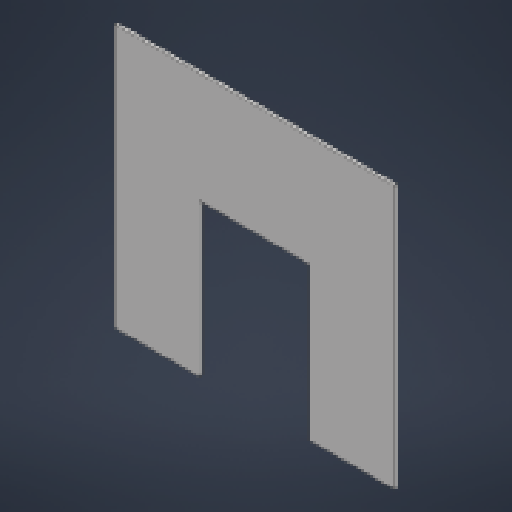
# Autodesk Inventor part: второй верх
Saved by Autodesk Inventor 2026.2 (Build 302298000, 298)
## iProperties
Created: 2025-11-21
Part Number: второй верх
Material: Типовые
Document SubType Name: Modeling
Designer: Phantom
Density: 1 g/cm^3
Appearance: По умолчанию
Author: Phantom
Autodesk Inventor part; units mm, degrees
ref_plane "YZ Plane" through (0, 0, 0) normal (1, 0, 0) x (0, 1, 0)
ref_plane "XZ Plane" through (0, 0, 0) normal (0, 1, 0) x (-1, 0, 0)
ref_plane "XY Plane" through (0, 0, 0) normal (0, 0, 1) x (1, 0, 0)
sketch "Эскиз1" plane through (0, 0, 0) normal (0, 0, 1) x (1, 0, 0)
  line L0 (-202.5, -190) -> (202.5, -190)
  line L1 (202.5, -190) -> (202.5, 190)
  line L2 (202.5, 190) -> (-202.5, 190)
  line L3 (-202.5, 190) -> (-202.5, -190)
  line L4 (-202.5, -190) -> (202.5, 190) construction
  line L5 (202.5, -190) -> (-202.5, 190) construction
  point P0 (0, 0)
  dimension "d0" = 405
  dimension "d1" = 380
  constraints: 12 end point, 2 midpoint, 2 parallel, 1 horizontal, 1 perpendicular
  measures "d0" distance of L2.end L1.end
  measures "d1" distance of L1.end L0.end
extrude "Выдавливание1" add sketch "Эскиз1" along normal blind 4
sketch "Эскиз2" plane through (0, 0, 4) normal (0, 0, 1) x (1, 0, 0)
  line L0 (-202.5, -190) -> (202.5, -190) projected
  line L1 (0, -190) -> (0, 30)
  line L2 (-80, 30) -> (80, 30)
  line L3 (80, 30) -> (80, -190)
  line L4 (80, -190) -> (-80, -190)
  line L5 (-80, -190) -> (-80, 30)
  line L6 (-80, 30) -> (80, -190) construction
  line L7 (80, 30) -> (-80, -190) construction
  point P0 (0, 0)
  point P1 (0, -80)
  dimension "d4" = 220
  dimension "d5" = 160
  constraints: 14 end point, 4 midpoint, 2 parallel, 1 horizontal, 1 perpendicular, 1 point on line, 1 vertical
  measures "d4" distance of L1.start L1.end
  measures "d5" distance of L2.start L2.end
extrude "Выдавливание2" cut sketch "Эскиз2" against normal blind 10
